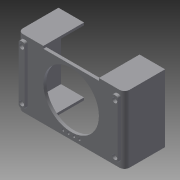
# Autodesk Inventor part: Enclosure01
Saved by Autodesk Inventor 2013 (Build 170138000, 138)
## iProperties
Created: 2014-04-13
Part Number: Enclosure01
Material: Generic
Document SubType Name: Modeling
Designer: spichelh
Density: 1 g/cm^3
Author: spichelh
Autodesk Inventor part; units mm, degrees
ref_plane "YZ Plane" through (0, 0, 0) normal (1, 0, 0) x (0, 1, 0)
ref_plane "XZ Plane" through (0, 0, 0) normal (0, 1, 0) x (-1, 0, 0)
ref_plane "XY Plane" through (0, 0, 0) normal (0, 0, 1) x (1, 0, 0)
sketch "Sketch1" plane through (0, 0, 0) normal (0, 0, 1) x (1, 0, 0)
  circle A0 centre (31.4469, 31.0185) radius 28
  line L0 (-19.3531, 3.1035) -> (82.2469, 3.1035) construction
  line L1 (8.4469, 60.2535) -> (-19.3531, 60.2535) construction
  line L2 (82.2469, 60.2535) -> (54.3269, 60.2535) construction
  line L3 (82.2469, 3.1035) -> (82.2469, 60.2535) construction
  line L4 (-19.3531, 60.2535) -> (-19.3531, 3.1035) construction
  line L5 (5.509, 60.2207) -> (61.389, 60.2207) construction
  line L6 (61.389, 60.2207) -> (61.389, 72.2207) construction
  line L7 (61.389, 72.2207) -> (5.509, 72.2207) construction
  line L8 (5.509, 72.2207) -> (5.509, 60.2207) construction
  circle A1 centre (61.389, 6.2635) radius 1.5 construction
  circle A2 centre (61.389, 55.7935) radius 1.5 construction
  circle A3 centre (5.509, 55.7935) radius 1.5 construction
  circle A4 centre (5.509, 6.9135) radius 1.5 construction
  arc A5 (5.509, 7.6907) -> (5.509, 1.6907) centre (5.509, 4.6907) ccw construction
  line L9 (5.509, 1.6907) -> (5.509, -3.7465) construction
  line L10 (5.509, -3.7465) -> (61.389, -3.7465) construction
  line L11 (61.389, -3.7465) -> (61.389, 1.6907) construction
  arc A6 (61.389, 1.6907) -> (61.389, 7.6907) centre (61.389, 4.6907) ccw construction
  line L12 (61.389, 7.6907) -> (61.389, 51.2207) construction
  arc A7 (61.389, 51.2207) -> (61.389, 57.2207) centre (61.389, 54.2207) ccw construction
  line L13 (61.389, 57.2207) -> (61.389, 60.2207) construction
  line L14 (61.389, 60.2207) -> (5.509, 60.2207) construction
  line L15 (5.509, 60.2207) -> (5.509, 57.2207) construction
  arc A8 (5.509, 57.2207) -> (5.509, 51.2207) centre (5.509, 54.2207) ccw construction
  line L16 (5.509, 51.2207) -> (5.509, 7.6907) construction
  line L17 (-22.3531, -3.7465) -> (85.2469, -3.7465)
  line L18 (85.2469, -3.7465) -> (85.2469, 64.2535)
  line L19 (85.2469, 64.2535) -> (-22.3531, 64.2535)
  line L20 (-22.3531, 64.2535) -> (-22.3531, -3.7465)
  line L21 (31.4469, -3.7465) -> (31.4469, 64.2535) construction
  circle A9 centre (31.4469, 31.0185) radius 23 projected
  point P0 (0, 0)
  dimension "d42" = 0
  dimension "d43" = 3
  dimension "d44" = 3
  dimension "d45" = 4
  dimension "d46" = 4
  dimension "d47" = 57.15
  dimension "d48" = 57.15
  dimension "d49" = 101.6
  dimension "d50" = 3.81
  dimension "d56" = 68
  dimension "d59" = 56
  constraints: 44 end point, 9 centre point, 8 point on circle, 2 midpoint, 2 parallel, 1 concentric, 1 horizontal, 1 perpendicular, 1 point on line
  measures "d42" distance between parallel lines of L17 L10
  measures "d43" distance between parallel lines of L4 L20
  measures "d44" distance between parallel lines of L18 L3
  measures "d45" distance between parallel lines of L19 L1
  measures "d46" distance between parallel lines of L19 L2
  measures "d47" distance between parallel lines of L0 L1
  measures "d48" distance between parallel lines of L2 L0
  measures "d49" distance between parallel lines of L4 L3
  measures "d50" distance from line of L0 A4.centre
  measures "d56" distance between parallel lines of L19 L17
  measures "d59" diameter of A0
extrude "Extrusion1" add sketch "Sketch1" along normal blind 3 contours L20 L19 L18 L17
sketch "Sketch2" plane through (0, 0, 0) normal (0, 0, -1) x (-1, 0, 0)
  circle A0 centre (-31.4469, 31.0185) radius 28 projected
  line L0 (22.3531, -3.7465) -> (-85.2469, -3.7465) projected
  line L1 (22.3531, 64.2535) -> (22.3531, -3.7465) projected
  line L2 (-85.2469, 64.2535) -> (22.3531, 64.2535) projected
  line L3 (-85.2469, -3.7465) -> (-85.2469, 64.2535) projected
  line L4 (-82.7469, 61.7535) -> (19.8531, 61.7535)
  line L5 (19.8531, 61.7535) -> (19.8531, -1.2465)
  line L6 (19.8531, -1.2465) -> (-82.7469, -1.2465)
  line L7 (-82.7469, -1.2465) -> (-82.7469, 61.7535)
  dimension "d51" = 2.5
  dimension "d52" = 2.5
  dimension "d53" = 2.5
  dimension "d54" = 2.5
  constraints: 8 end point, 2 parallel, 1 horizontal, 1 perpendicular
  measures "d51" distance between parallel lines of L4 L2
  measures "d52" distance between parallel lines of L3 L7
  measures "d53" distance between parallel lines of L1 L5
  measures "d54" distance between parallel lines of L0 L6
extrude "Extrusion2" add sketch "Sketch2" along normal blind 38 contours L0 L3 L2 L1
sketch "Sketch4" plane through (0, 0, 3) normal (0, 0, 1) x (1, 0, 0)
  circle A0 centre (-15.5431, 55.7835) radius 1.5 projected
  circle A1 centre (-15.5431, 6.2535) radius 1.5 projected
  circle A2 centre (78.4369, 6.2535) radius 1.5 projected
  circle A3 centre (78.4369, 55.7835) radius 1.5 projected
  point P0 (0, 0)
extrude "Extrusion3" cut sketch "Sketch4" against normal blind 3
chamfer "Chamfer1" [suppressed]
sketch "Sketch5" plane through (-22.3531, 64.2535, 3) normal (0, 1, 0) x (1, 0, 0)
  line L0 (0, 0) -> (107.6, 0)
  line L1 (25.8, 63) -> (81.8, 63)
  line L2 (81.8, 63) -> (81.8, 7)
  line L3 (81.8, 7) -> (25.8, 7)
  line L4 (25.8, 7) -> (25.8, 63)
  line L5 (53.8, 0) -> (53.8, -31.7336) construction
  line L6 (25.8, 63) -> (81.8, 7) construction
  line L7 (81.8, 63) -> (25.8, 7) construction
  line L8 (104.9242, 0) -> (-0.6758, 0)
  line L9 (107.6, 0) -> (0, 0) projected
  line L10 (0, 41) -> (107.6, 41) projected
  line L11 (53.8, 41) -> (53.8, 0) construction
  point P0 (19.351, -30)
  point P1 (53.8, 35)
  point P2 (53.8, 35)
  dimension "d28" = 56
  dimension "d29" = 56
  dimension "d41" = 7
  constraints: 20 end point, 5 midpoint, 3 parallel, 2 point on line, 1 collinear, 1 horizontal, 1 perpendicular
  measures "d28" distance of L2.end L3.end
  measures "d29" distance of L1.end L2.end
  measures "d41" distance between parallel lines of L8 L3
extrude "Extrusion4" cut sketch "Sketch5" against normal blind 100
fillet "Fillet2" radius 5 2 edges at (-22.3531, 30.2535, 3) (85.2469, 30.2535, 3)
fillet "Fillet3" radius 5 2 edges at (-19.8531, 30.2535, 0) (82.7469, 30.2535, 0)
sketch "Sketch6" plane through (3.4469, 64.2535, -4) normal (0, 1, 0) x (1, 0, 0)
  line L0 (76.8, -7) -> (-20.8, -7) projected
  line L1 (0, 0) -> (56, 0)
  line L2 (56, 0) -> (56, -7)
  line L3 (56, -7) -> (0, -7)
  line L4 (0, -7) -> (0, 0)
  point P0 (-3.4469, -4)
  constraints: 8 end point, 2 parallel, 1 horizontal, 1 perpendicular, 1 point on line
extrude "Extrusion5" cut sketch "Sketch6" against normal blind 2.5
sketch "Sketch7" plane through (0, 0, 3) normal (0, 0, 1) x (1, 0, 0)
  line L0 (-17.3531, -3.7465) -> (80.2469, -3.7465) projected
  line L1 (59.4469, 61.7535) -> (3.4469, 61.7535) projected
  line L2 (31.4469, -3.7465) -> (31.4469, 61.7535) construction
  line L3 (23.1969, -0.7465) -> (23.1969, -0.7465)
  line L4 (22.1969, 0.2535) -> (22.1969, 1.2535)
  line L5 (23.1969, 2.2535) -> (23.1969, 2.2535)
  line L6 (24.1969, 1.2535) -> (24.1969, 0.2535)
  arc A0 (24.1969, 1.2535) -> (23.1969, 2.2535) centre (23.1969, 1.2535) ccw
  arc A1 (23.1969, 2.2535) -> (22.1969, 1.2535) centre (23.1969, 1.2535) ccw
  arc A2 (22.1969, 0.2535) -> (23.1969, -0.7465) centre (23.1969, 0.2535) ccw
  arc A3 (23.1969, -0.7465) -> (24.1969, 0.2535) centre (23.1969, 0.2535) ccw
  line L7 (27.6969, 0.2535) -> (27.6969, 1.2535)
  line L8 (29.6969, 1.2535) -> (29.6969, 0.2535)
  arc A4 (29.6969, 1.2535) -> (28.6969, 2.2535) centre (28.6969, 1.2535) ccw
  arc A5 (28.6969, 2.2535) -> (27.6969, 1.2535) centre (28.6969, 1.2535) ccw
  arc A6 (27.6969, 0.2535) -> (28.6969, -0.7465) centre (28.6969, 0.2535) ccw
  arc A7 (28.6969, -0.7465) -> (29.6969, 0.2535) centre (28.6969, 0.2535) ccw
  line L9 (33.1969, 0.2535) -> (33.1969, 1.2535)
  line L10 (35.1969, 1.2535) -> (35.1969, 0.2535)
  arc A8 (35.1969, 1.2535) -> (34.1969, 2.2535) centre (34.1969, 1.2535) ccw
  arc A9 (34.1969, 2.2535) -> (33.1969, 1.2535) centre (34.1969, 1.2535) ccw
  arc A10 (33.1969, 0.2535) -> (34.1969, -0.7465) centre (34.1969, 0.2535) ccw
  arc A11 (34.1969, -0.7465) -> (35.1969, 0.2535) centre (34.1969, 0.2535) ccw
  line L11 (38.6969, 0.2535) -> (38.6969, 1.2535)
  line L12 (40.6969, 1.2535) -> (40.6969, 0.2535)
  arc A12 (40.6969, 1.2535) -> (39.6969, 2.2535) centre (39.6969, 1.2535) ccw
  arc A13 (39.6969, 2.2535) -> (38.6969, 1.2535) centre (39.6969, 1.2535) ccw
  arc A14 (38.6969, 0.2535) -> (39.6969, -0.7465) centre (39.6969, 0.2535) ccw
  arc A15 (39.6969, -0.7465) -> (40.6969, 0.2535) centre (39.6969, 0.2535) ccw
  line L13 (29.6969, 0.7535) -> (33.1969, 0.7535) construction
  point P0 (0, 0)
  point P1 (24.1969, -0.7465)
  point P2 (22.1969, 2.2535)
  point P3 (24.1969, 2.2535)
  point P4 (29.6969, -0.7465)
  point P5 (27.6969, 2.2535)
  point P6 (29.6969, 2.2535)
  point P7 (35.1969, -0.7465)
  point P8 (33.1969, 2.2535)
  point P9 (35.1969, 2.2535)
  point P10 (40.6969, -0.7465)
  point P11 (38.6969, 2.2535)
  point P12 (40.6969, 2.2535)
  point P13 (31.4469, 0.7535)
  dimension "d64" = 2
  dimension "d66" = 3
  dimension "d67" = 1
  dimension "d68" = 1
  dimension "d69" = 4
  dimension "d78" = 16.5
  dimension "d79" = 7.25
  dimension "d80" = 7.25
  constraints: 32 point on circle, 24 end point, 16 centre point, 16 point on line, 8 tangent, 5 midpoint, 2 equal radius, 2 parallel, 1 horizontal, 1 perpendicular
  measures "d64" distance of point (22.197, 2.253) point (24.197, 2.253)
  measures "d66" distance of point (24.197, 2.253) point (24.197, -0.747)
  measures "d67" radius of A0
  measures "d68" radius of A3
  measures "d69" distance from line of L0 A3.centre
  measures "d78" distance of A14.centre A3.centre
  measures "d79" distance from line of L6 point (31.447, 0.753)
  measures "d80" distance from line of point (31.447, 0.753) L11
extrude "Extrusion6" cut sketch "Sketch7" against normal blind 3
sketch "Sketch10" plane through (0, 0, 3) normal (0, 0, 1) x (1, 0, 0)
  circle A0 centre (31.4469, 31.0185) radius 28 projected
  circle A1 centre (78.4369, 55.7835) radius 1.5 projected
  circle A2 centre (-15.5431, 6.2535) radius 1.5 projected
  circle A3 centre (-15.5431, 55.7835) radius 1.5 projected
  circle A4 centre (78.4369, 6.2535) radius 1.5 projected
  line L0 (-14.5431, 60.2835) -> (-16.5431, 60.2835)
  line L1 (-18.5431, 58.2835) -> (-18.5431, 3.7535)
  line L2 (-16.5431, 1.7535) -> (-14.5431, 1.7535)
  line L3 (-12.5431, 3.7535) -> (-12.5431, 58.2835)
  arc A5 (-12.5431, 58.2835) -> (-14.5431, 60.2835) centre (-14.5431, 58.2835) ccw
  arc A6 (-16.5431, 60.2835) -> (-18.5431, 58.2835) centre (-16.5431, 58.2835) ccw
  arc A7 (-14.5431, 1.7535) -> (-12.5431, 3.7535) centre (-14.5431, 3.7535) ccw
  arc A8 (-18.5431, 3.7535) -> (-16.5431, 1.7535) centre (-16.5431, 3.7535) ccw
  line L4 (31.4469, 31.0185) -> (31.4469, 47.569) construction
  line L5 (77.4369, 60.2835) -> (79.4369, 60.2835)
  line L6 (81.4369, 58.2835) -> (81.4369, 3.7535)
  line L7 (79.4369, 1.7535) -> (77.4369, 1.7535)
  line L8 (75.4369, 3.7535) -> (75.4369, 58.2835)
  arc A9 (77.4369, 60.2835) -> (75.4369, 58.2835) centre (77.4369, 58.2835) ccw
  arc A10 (81.4369, 58.2835) -> (79.4369, 60.2835) centre (79.4369, 58.2835) ccw
  arc A11 (75.4369, 3.7535) -> (77.4369, 1.7535) centre (77.4369, 3.7535) ccw
  arc A12 (79.4369, 1.7535) -> (81.4369, 3.7535) centre (79.4369, 3.7535) ccw
  point P0 (0, 0)
  dimension "d101" = 3
  dimension "d103" = 3
  dimension "d104" = 3
  dimension "d105" = 3
  dimension "d106" = 2
  dimension "d107" = 2
  constraints: 18 end point, 16 point on circle, 12 symmetric about line, 8 centre point, 8 tangent, 3 parallel, 2 equal radius, 1 horizontal, 1 perpendicular, 4 other
  measures "d101" distance edge to line of A2 L2
  measures "d103" distance edge to line of A3 L0
  measures "d104" distance from line of L1 A2.centre
  measures "d105" distance from line of L3 A3.centre
  measures "d106" radius of A5
  measures "d107" radius of A6
extrude "Extrusion9" add sketch "Sketch10" along normal blind 3 and the other way blind 2 contours A5 L3 A7 L2 A8 L1 A6 L0 | L5 A10 L6 A12 L7 A11 L8 A9
sketch "Sketch11" plane through (0, 0, 6) normal (0, 0, 1) x (1, 0, 0)
  circle A0 centre (-15.5431, 55.7835) radius 1.5 projected
  circle A1 centre (-15.5431, 6.2535) radius 1.5 projected
  circle A2 centre (78.4369, 6.2535) radius 1.5 projected
  circle A3 centre (78.4369, 55.7835) radius 1.5 projected
  line L0 (75.4369, 58.2835) -> (75.4369, 3.7535) projected
  arc A4 (75.4369, 3.7535) -> (77.4369, 1.7535) centre (77.4369, 3.7535) ccw projected
  line L1 (77.4369, 1.7535) -> (79.4369, 1.7535) projected
  arc A5 (79.4369, 1.7535) -> (81.4369, 3.7535) centre (79.4369, 3.7535) ccw projected
  line L2 (81.4369, 3.7535) -> (81.4369, 58.2835) projected
  arc A6 (81.4369, 58.2835) -> (79.4369, 60.2835) centre (79.4369, 58.2835) ccw projected
  line L3 (79.4369, 60.2835) -> (77.4369, 60.2835) projected
  arc A7 (77.4369, 60.2835) -> (75.4369, 58.2835) centre (77.4369, 58.2835) ccw projected
  circle A8 centre (-15.5431, 55.7835) radius 2.5
  circle A9 centre (-15.5431, 6.2535) radius 2.5
  circle A10 centre (78.4369, 55.7835) radius 2.5
  circle A11 centre (78.4369, 6.2535) radius 2.5
  point P0 (0, 0)
  dimension "d112" = 5
  dimension "d114" = 5
  dimension "d115" = 5
  dimension "d116" = 5
  constraints: 4 centre point
  measures "d112" diameter of A8
  measures "d114" diameter of A9
  measures "d115" diameter of A10
  measures "d116" diameter of A11
extrude "Extrusion10" cut sketch "Sketch11" against normal blind 3 contours A0 | A1 | A2 | A3 | A8 | A9 | A10 | A11
body "Solid1"
